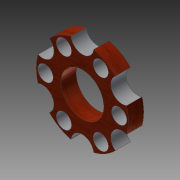
# Autodesk Inventor part: Статор цевков
Saved by Autodesk Inventor 2013 (Build 170138000, 138)
## iProperties
Created: 2014-04-30
Part Number: Статор цевков
Material: Типовые
Document SubType Name: Modeling
Designer: HP1
Density: 1 g/cm^3
Author: HP1
Autodesk Inventor part; units mm, degrees
ref_plane "YZ Plane" through (0, 0, 0) normal (1, 0, 0) x (0, 1, 0)
ref_plane "XZ Plane" through (0, 0, 0) normal (0, 1, 0) x (-1, 0, 0)
ref_plane "XY Plane" through (0, 0, 0) normal (0, 0, 1) x (1, 0, 0)
sketch "Эскиз1" plane through (0, 0, 0) normal (0, 1, 0) x (-1, 0, 0)
  circle A0 centre (0, 0) radius 14
  circle A1 centre (0, 0) radius 24 construction
  circle A2 centre (0, 0) radius 30
  circle A3 centre (23.9999, 0) radius 5
  circle A4 centre (12, 20.7845) radius 5
  circle A5 centre (-12, 20.7845) radius 5
  circle A6 centre (-23.9999, 0) radius 5
  circle A7 centre (-12, -20.7845) radius 5
  circle A8 centre (12, -20.7845) radius 5
  dimension "d0" = 28
  dimension "d1" = 48
  dimension "d2" = 60
  dimension "d3" = 10
  dimension "d6" = 360
  constraints: 9 centre point, 13 other
  measures "d0" diameter of A0
  measures "d1" diameter of A1
  measures "d2" diameter of A2
  measures "d3" diameter of A3
extrude "Выдавливание1" add sketch "Эскиз1" along normal blind 10
sketch "Эскиз2" plane through (0, 10, 0) normal (0, 1, 0) x (1, 0, 0)
  circle A0 centre (0, 0) radius 14 projected
  circle A1 centre (0, 29.9993) radius 7.5
  circle A2 centre (-25.9801, 14.9996) radius 7.5
  circle A3 centre (-25.9801, -14.9996) radius 7.5
  circle A4 centre (0, -29.9993) radius 7.5
  circle A5 centre (25.9801, -14.9996) radius 7.5
  circle A6 centre (25.9801, 14.9996) radius 7.5
  dimension "d10" = 15
  dimension "d13" = 360
  constraints: 6 centre point, 13 other
  measures "d10" diameter of A1
extrude "Выдавливание2" cut sketch "Эскиз2" against normal blind 10 contours A1 | A2 | A3 | A4 | A5 | A6
